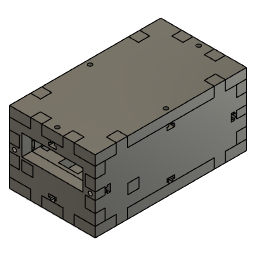
Basic-Case_v1 (Autodesk Fusion 360 design; units mm, degrees)
Autodesk Fusion 360 part; units mm, degrees
(part 1 of 2)
ref_plane "WorkPlane4" through (0, 21, 0) normal (0, 1, 0) x (0, 0, 1)
ref_plane "WorkPlane5" through (0, 0, 26.5) normal (0, 0, 1) x (1, 0, 0)
ref_plane "WorkPlane9" through (0, 0, -26.5) normal (0, 0, 1) x (1, 0, 0)
ref_plane "WorkPlane11" through (-13.285, 0, 0) normal (1, 0, 0) x (0, 1, 0)
ref_plane "WorkPlane12" through (13.285, 0, 0) normal (1, 0, 0) x (0, 1, 0)
sketch "Sketch1" plane through (0, 0, 0) normal (0, 1, 0) x (1, 0, 0)
  line L0 (12.785, -26) -> (-12.785, -26) construction
  line L1 (-12.785, -26) -> (-12.785, 26) construction
  line L2 (-12.785, 26) -> (12.785, 26) construction
  line L3 (12.785, 26) -> (12.785, -26) construction
  line L4 (12.785, -26) -> (-12.785, 26) construction
  line L5 (-12.785, -26) -> (12.785, 26) construction
  line L6 (-13.285, -26.5) -> (-13.285, 26.5)
  line L7 (-13.285, 26.5) -> (13.285, 26.5)
  line L8 (13.285, 26.5) -> (13.285, -26.5)
  line L9 (13.285, -26.5) -> (-13.285, -26.5)
  line L10 (-17.285, -30.5) -> (-17.285, 30.5)
  line L11 (-17.285, 30.5) -> (17.285, 30.5)
  line L12 (17.285, 30.5) -> (17.285, -30.5)
  line L13 (17.285, -30.5) -> (-17.285, -30.5)
  line L14 (-17.285, -22) -> (-12.785, -22)
  line L15 (-17.285, -17.5) -> (-13.285, -17.5)
  line L16 (-8.785, -26.5) -> (-8.785, -30.5)
  line L17 (-4.285, -30.5) -> (-4.285, -26.5)
  line L18 (4.285, -26.5) -> (4.285, -30.5)
  line L19 (8.785, -30.5) -> (8.785, -26.5)
  line L20 (13.285, -22) -> (17.285, -22)
  line L21 (13.285, -17.5) -> (17.285, -17.5)
  line L22 (13.285, 22) -> (17.285, 22)
  line L23 (17.285, 17.5) -> (13.285, 17.5)
  line L24 (8.785, 30.5) -> (8.785, 26.5)
  line L25 (4.285, 30.5) -> (4.285, 26.5)
  line L26 (-8.785, 30.5) -> (-8.785, 26.5)
  line L27 (-4.285, 26.5) -> (-4.285, 30.5)
  line L28 (-13.285, 22) -> (-17.285, 22)
  line L29 (-17.285, 17.5) -> (-13.285, 17.5)
  line L30 (0, -26.5) -> (0, -30.5) construction
  line L31 (13.285, 0) -> (17.285, 0) construction
  line L32 (-17.285, 0) -> (-13.285, 0) construction
  line L33 (0, 30.5) -> (0, 26.5) construction
  circle A0 centre (15.285, 0) radius 0.8
  circle A1 centre (0, 28.5) radius 0.8
  circle A2 centre (-15.285, 0) radius 0.8
  circle A3 centre (0, -28.5) radius 0.8
  dimension "d1" = 52
  dimension "d2" = 25.57
  dimension "d3" = 0.5
  dimension "d4" = 4.5
  dimension "d385" = 4.5
  dimension "d386" = 4.5
  dimension "d387" = 4.5
  dimension "d388" = 4.5
  dimension "d389" = 4.5
  dimension "d391" = 4.5
  dimension "d392" = 4.5
  dimension "d394" = 4.5
  dimension "d395" = 4.5
  dimension "d396" = 4.5
  dimension "d397" = 4.5
  dimension "d399" = 4.5
  dimension "d402" = 1.6
  dimension "d403" = 1.6
  dimension "d404" = 1.6
  dimension "d405" = 1.6
  dimension "d437" = 4.5
  dimension "d438" = 4.5
  dimension "d439" = 4.5
  dimension "d440" = 4.5
  constraint perpendicular L0 L1
  constraint parallel L0 L2
  constraint parallel L1 L3
  constraint horizontal L0
  constraint coincident L4 origin
  constraint coincident L5 origin
  constraint coincident L10 L14.start
  constraint coincident L1 L14.end
  constraint perpendicular L6 L14
  constraint coincident L10 L15.start
  constraint coincident L6 L15.end
  constraint perpendicular L1 L15
  constraint coincident L9 L16.start
  constraint coincident L13 L16.end
  constraint perpendicular L13 L16
  constraint coincident L13 L17.start
  constraint coincident L9 L17.end
  constraint perpendicular L9 L17
  constraint coincident L9 L18.start
  constraint coincident L13 L18.end
  constraint perpendicular L13 L18
  constraint coincident L13 L19.start
  constraint coincident L9 L19.end
  constraint perpendicular L0 L19
  constraint coincident L8 L20.start
  constraint coincident L12 L20.end
  constraint perpendicular L12 L20
  constraint coincident L8 L21.start
  constraint coincident L12 L21.end
  constraint perpendicular L12 L21
  constraint coincident L8 L22.start
  constraint coincident L12 L22.end
  constraint perpendicular L12 L22
  constraint coincident L12 L23.start
  constraint coincident L8 L23.end
  constraint perpendicular L8 L23
  constraint coincident L11 L24.start
  constraint coincident L7 L24.end
  constraint perpendicular L7 L24
  constraint coincident L11 L25.start
  constraint coincident L7 L25.end
  constraint perpendicular L11 L25
  constraint coincident L11 L26.start
  constraint coincident L7 L26.end
  constraint perpendicular L7 L26
  constraint coincident L7 L27.start
  constraint coincident L11 L27.end
  constraint perpendicular L11 L27
  constraint coincident L6 L28.start
  constraint coincident L10 L28.end
  constraint perpendicular L10 L28
  constraint coincident L10 L29.start
  constraint coincident L6 L29.end
  constraint perpendicular L6 L29
  constraint midpoint L9 L30.start
  constraint midpoint L13 L30.end
  constraint midpoint L8 L31.start
  constraint midpoint L12 L31.end
  constraint midpoint L10 L32.start
  constraint midpoint L6 L32.end
  constraint midpoint L11 L33.start
  constraint midpoint L7 L33.end
  constraint midpoint L31 A0.centre
  constraint midpoint L33 A1.centre
  constraint midpoint L32 A2.centre
  constraint midpoint L30 A3.centre
  measures "d1" distance of L0.start L2.end
  measures "d2" distance of L0.start L0.end
  measures "d385" distance of L28 L29
  measures "d386" distance of L26 L27
  measures "d387" distance of L6.end L26
  measures "d388" distance of L24 L25
  measures "d389" distance of L7.end L24
  measures "d391" distance of L22 L23
  measures "d392" distance of L20 L21
  measures "d394" distance of L8.end L19
  measures "d395" distance of L18 L19
  measures "d396" distance of L6.start L16
  measures "d397" distance of L16 L17
  measures "d402" diameter of A3
  measures "d403" diameter of A0
  measures "d404" diameter of A2
  measures "d405" diameter of A1
  measures "d437" distance of L6.start L14
  measures "d438" distance of L6.end L28
  measures "d439" distance of L7.end L22
  measures "d440" distance of L8.end L20
sketch "Sketch33" plane through (0, 21, 0) normal (0, 1, 0) x (1, 0, 0)
  line L0 (-17.285, 30.5) -> (17.285, 30.5)
  line L1 (-17.285, -30.5) -> (-17.285, 30.5)
  line L2 (17.285, -30.5) -> (-17.285, -30.5)
  line L3 (-13.285, -26.5) -> (-13.285, 26.5)
  line L4 (-13.285, 26.5) -> (13.285, 26.5)
  line L5 (-13.285, 22) -> (-17.285, 22)
  line L6 (-17.285, 17.5) -> (-13.285, 17.5)
  line L7 (-8.785, 30.5) -> (-8.785, 26.5)
  line L8 (-4.285, 26.5) -> (-4.285, 30.5)
  line L9 (4.285, 30.5) -> (4.285, 26.5)
  line L10 (8.785, 30.5) -> (8.785, 26.5)
  line L11 (13.285, 26.5) -> (13.285, -26.5)
  line L12 (13.285, 22) -> (17.285, 22)
  line L13 (17.285, 17.5) -> (13.285, 17.5)
  line L14 (17.285, 30.5) -> (17.285, -30.5)
  line L15 (13.285, -17.5) -> (17.285, -17.5)
  line L16 (13.285, -22) -> (17.285, -22)
  line L17 (8.785, -30.5) -> (8.785, -26.5)
  line L18 (4.285, -26.5) -> (4.285, -30.5)
  line L19 (-4.285, -30.5) -> (-4.285, -26.5)
  line L20 (-8.785, -26.5) -> (-8.785, -30.5)
  line L21 (-17.285, -22) -> (-12.785, -22)
  line L22 (-17.285, -17.5) -> (-13.285, -17.5)
  line L23 (13.285, -26.5) -> (-13.285, -26.5)
  circle A0 centre (0, -28.5) radius 0.8
  circle A1 centre (0, 28.5) radius 0.8
  circle A2 centre (-15.285, 0) radius 0.8
  circle A3 centre (15.285, 0) radius 0.8
  point P0 (15.285, 0)
  point P1 (-15.285, 0)
sketch "Sketch24" plane through (0, 0, 26.5) normal (0, 0, 1) x (1, 0, 0)
  line L0 (17.285, 0) -> (-17.285, 0)
  line L1 (17.285, 21) -> (-17.285, 21)
  line L2 (-8.785, 21) -> (-8.785, 25)
  line L3 (-4.285, 21) -> (-4.285, 25)
  line L4 (4.285, 21) -> (4.285, 25)
  line L5 (8.785, 21) -> (8.785, 25)
  line L6 (-8.785, 0) -> (-8.785, -4)
  line L7 (-4.285, 0) -> (-4.285, -4)
  line L8 (4.285, 0) -> (4.285, -4)
  line L9 (8.785, 0) -> (8.785, -4)
  line L10 (-0.8, 21) -> (-0.8, 20.1)
  line L11 (-0.8, 20.1) -> (-1.5, 20.1)
  line L12 (-1.5, 20.1) -> (-1.5, 18.9)
  line L13 (-1.5, 18.9) -> (1.5, 18.9)
  line L14 (1.5, 18.9) -> (1.5, 20.1)
  line L15 (1.5, 20.1) -> (0.8, 20.1)
  line L16 (0.8, 20.1) -> (0.8, 21)
  line L17 (-0.8, 0) -> (-0.8, 0.9)
  line L18 (-1.5, 0.9) -> (-1.5, 2.1)
  line L19 (-1.5, 2.1) -> (1.5, 2.1)
  line L20 (-0.8, 0.9) -> (-1.5, 0.9)
  line L21 (1.5, 0.9) -> (0.8, 0.9)
  line L22 (0.8, 0.9) -> (0.8, 0)
  line L23 (1.5, 2.1) -> (1.5, 0.9)
  line L24 (0, 18.9) -> (0, 21) construction
  line L25 (0, 2.1) -> (0, 0) construction
  line L26 (13.285, 16.5) -> (24.3607, 16.5)
  line L27 (13.285, 4.5) -> (17.285, 4.5)
  line L28 (-13.285, 12) -> (-17.285, 12)
  line L29 (-17.285, 9) -> (-13.285, 9)
  line L30 (-17.285, 25) -> (-17.285, -4)
  line L31 (-17.285, -4) -> (17.285, -4)
  line L32 (17.285, -4) -> (17.285, 25)
  line L33 (17.285, 25) -> (-17.285, 25)
  line L34 (-13.285, 21) -> (-13.285, 0)
  line L35 (13.285, 21) -> (13.285, 0)
  line L36 (17.285, 9) -> (13.285, 9)
  line L37 (17.285, 12) -> (13.285, 12)
  line L38 (-13.285, 16.5) -> (-17.285, 16.5)
  line L39 (-13.285, 4.5) -> (-17.285, 4.5)
  line L40 (17.285, 10.5) -> (13.285, 10.5) construction
  line L41 (-13.285, 10.5) -> (-13.285, 14.6467)
  line L42 (-17.285, 10.5) -> (-13.285, 10.5) construction
  circle A0 centre (15.285, 10.5) radius 0.8
  circle A1 centre (-15.285, 10.5) radius 0.8
  line L43 (0, 0) -> (0, 25) construction
  point P0 (-4.285, 0)
  point P1 (-8.785, 0)
  point P2 (4.285, 0)
  point P3 (8.785, 0)
  point P4 (0, 21)
  point P5 (-8.785, 21)
  point P6 (-4.285, 21)
  point P7 (8.785, 21)
  point P8 (4.285, 21)
  dimension "d406" = 3
  dimension "d407" = 1.2
  dimension "d409" = 1.6
  dimension "d410" = 1.6
  dimension "d411" = 3
  dimension "d413" = 1.2
  dimension "d420" = 6.1
  dimension "d421" = 4
  dimension "d422" = 4
  dimension "d424" = 6.1
  dimension "d425" = 4
  dimension "d426" = 4
  dimension "d427" = 4.5
  dimension "d428" = 4.5
  dimension "d429" = 4.5
  dimension "d430" = 4.5
  dimension "d433" = 4.5
  dimension "d434" = 4.5
  dimension "d435" = 1.6
  dimension "d436" = 1.6
  dimension "d482" = 4.5
  dimension "d483" = 4.5
  constraint coincident P1 L6.start
  constraint coincident P0 L7.start
  constraint coincident P2 L8.start
  constraint perpendicular L0 L8
  constraint coincident P3 L9.start
  constraint perpendicular L10 L11
  constraint perpendicular L12 L13
  constraint perpendicular L14 L15
  constraint collinear L11 L15
  constraint equal L11 L15
  constraint equal L17 L22
  constraint equal L18 L23
  constraint equal L20 L21
  constraint perpendicular L18 L19
  constraint perpendicular L19 L23
  constraint perpendicular L18 L20
  constraint perpendicular L21 L22
  constraint midpoint L13 L24.start
  constraint coincident P4 L24.end
  constraint perpendicular L1 L24
  constraint midpoint L19 L25.start
  constraint coincident L25.end L43.start
  constraint perpendicular L0 L25
  constraint perpendicular L1 L3
  constraint perpendicular L1 L2
  constraint perpendicular L1 L4
  constraint perpendicular L1 L5
  constraint vertical L30
  constraint perpendicular L32 L33
  constraint perpendicular L30 L33
  constraint perpendicular L30 L31
  constraint coincident L2.end L33
  constraint coincident L3.end L33
  constraint coincident L4.end L33
  constraint coincident L5.end L33
  constraint coincident L1.start L32
  constraint coincident L1.end L30
  constraint coincident L6.end L31
  constraint coincident L7.end L31
  constraint coincident L0 L17.start
  constraint coincident L0 L22.end
  constraint coincident L1 L10.start
  constraint coincident L1 L16.end
  constraint coincident L8.end L31
  constraint coincident L9.end L31
  constraint coincident L1 L34.start
  constraint coincident L0 L34.end
  constraint perpendicular L0 L34
  constraint coincident L1 L35.start
  constraint coincident L0 L35.end
  constraint perpendicular L0 L35
  constraint coincident L28.start L34
  constraint coincident L29.end L34
  constraint coincident L26.start L35
  constraint coincident L27.start L35
  constraint perpendicular L0 L9
  constraint perpendicular L0 L6
  constraint perpendicular L0 L7
  constraint coincident L27.end L32
  constraint perpendicular L27 L32
  constraint coincident L32 L36.start
  constraint coincident L35 L36.end
  constraint perpendicular L35 L36
  constraint coincident L32 L37.start
  constraint coincident L35 L37.end
  constraint perpendicular L35 L37
  constraint coincident L34 L38.start
  constraint coincident L30 L38.end
  constraint perpendicular L30 L38
  constraint coincident L34 L39.start
  constraint coincident L30 L39.end
  constraint perpendicular L30 L39
  constraint coincident L29.start L30
  constraint perpendicular L29 L30
  constraint midpoint L32 L40.start
  constraint midpoint L35 L40.end
  constraint midpoint L34 L41.start
  constraint coincident L34 L41.end
  constraint parallel L34 L41
  constraint midpoint L30 L42.start
  constraint midpoint L40 A0.centre
  constraint midpoint L42 A1.centre
  constraint midpoint L33 L43.end
  constraint vertical L43
  constraint equal L12 L14
  constraint coincident L1 P8
  constraint coincident L1 P7
  constraint coincident L1 P6
  constraint coincident L1 P5
  constraint coincident P5 L2.start
  constraint coincident P6 L3.start
  constraint coincident P7 L5.start
  constraint coincident P8 L4.start
  constraint coincident L0.end L30
  constraint coincident L28.end L30
  measures "d406" distance of L12.end L13.end
  measures "d407" distance of L13.end L14.end
  measures "d409" distance of L10 L16
  measures "d410" distance of L17 L22
  measures "d411" horizontal distance of L18.end L19.end
  measures "d413" distance of L18.start L18.end
  measures "d420" distance of L13 L33
  measures "d421" distance of L1 L33
  measures "d422" distance of L0 L31
  measures "d424" distance of L19 L31
  measures "d425" distance of L30 L34
  measures "d426" distance of L32 L35
  measures "d427" distance of L28 L38
  measures "d428" distance of L29 L39
  measures "d429" distance of L26 L37
  measures "d430" distance of L27 L36
  measures "d433" distance of L0 L39
  measures "d434" distance of L0.start L27
  measures "d435" diameter of A1
  measures "d436" diameter of A0
  measures "d482" distance of L1 L38
  measures "d483" distance of L1 L26
sketch "Sketch38" plane through (0, 0, -26.5) normal (0, 0, 1) x (1, 0, 0)
  line L0 (17.285, 25) -> (-17.285, 25)
  line L1 (17.285, -4) -> (17.285, 25)
  line L2 (13.285, 21) -> (13.285, 0)
  line L3 (17.285, 21) -> (-17.285, 21)
  line L4 (8.785, 21) -> (8.785, 25)
  line L5 (4.285, 21) -> (4.285, 25)
  line L6 (-4.285, 21) -> (-4.285, 25)
  line L7 (-8.785, 21) -> (-8.785, 25)
  line L8 (0.8, 20.1) -> (0.8, 21)
  line L9 (1.5, 20.1) -> (0.8, 20.1)
  line L10 (1.5, 18.9) -> (1.5, 20.1)
  line L11 (-1.5, 18.9) -> (1.5, 18.9)
  line L12 (-1.5, 20.1) -> (-1.5, 18.9)
  line L13 (-0.8, 20.1) -> (-1.5, 20.1)
  line L14 (-0.8, 21) -> (-0.8, 20.1)
  line L15 (-13.285, 21) -> (-13.285, 0)
  line L16 (-17.285, 25) -> (-17.285, -4)
  line L17 (-13.285, 16.5) -> (-17.285, 16.5)
  line L18 (-13.285, 12) -> (-17.285, 12)
  circle A0 centre (-15.285, 10.5) radius 0.8
  line L19 (-17.285, 9) -> (-13.285, 9)
  line L20 (-13.285, 4.5) -> (-17.285, 4.5)
  line L21 (17.285, 0) -> (-17.285, 0)
  line L22 (-8.785, 0) -> (-8.785, -4)
  line L23 (-17.285, -4) -> (17.285, -4)
  line L24 (-4.285, 0) -> (-4.285, -4)
  line L25 (8.785, 0) -> (8.785, -4)
  line L26 (4.285, 0) -> (4.285, -4)
  line L27 (13.285, 4.5) -> (17.285, 4.5)
  line L28 (17.285, 9) -> (13.285, 9)
  circle A1 centre (15.285, 10.5) radius 0.8
  line L29 (17.285, 12) -> (13.285, 12)
  line L30 (13.285, 16.5) -> (24.3607, 16.5)
  line L31 (-1.5, 2.1) -> (1.5, 2.1)
  line L32 (1.5, 2.1) -> (1.5, 0.9)
  line L33 (1.5, 0.9) -> (0.8, 0.9)
  line L34 (-0.8, 0.9) -> (-1.5, 0.9)
  line L35 (-0.8, 0) -> (-0.8, 0.9)
  line L36 (0.8, 0.9) -> (0.8, 0)
  line L37 (-1.5, 0.9) -> (-1.5, 2.1)
sketch "Sketch39" plane through (13.285, 0, 0) normal (1, 0, 0) x (0, 1, 0)
  line L0 (21, -30.5) -> (21, 30.5)
  line L1 (0, -30.5) -> (0, 30.5)
  line L2 (-4, 26.5) -> (25, 26.5)
  line L3 (-4, -26.5) -> (25, -26.5)
  line L4 (25, 30.5) -> (25, -30.5)
  line L5 (25, -30.5) -> (-4, -30.5)
  line L6 (-4, -30.5) -> (-4, 30.5)
  line L7 (-4, 30.5) -> (25, 30.5)
  line L8 (21, 22) -> (25, 22)
  line L9 (21, 17.5) -> (25, 17.5)
  line L10 (21, -17.5) -> (25, -17.5)
  line L11 (21, -22) -> (25, -22)
  line L12 (16.5, -26.5) -> (16.5, -30.5)
  line L13 (12, -26.5) -> (12, -30.5)
  line L14 (9, -26.5) -> (9, -30.5)
  line L15 (4.5, -26.5) -> (4.5, -30.5)
  line L16 (0, -17.5) -> (-4, -17.5)
  line L17 (0, -22) -> (-4, -22)
  line L18 (0, 22) -> (-4, 22)
  line L19 (0, 17.5) -> (-4, 17.5)
  line L20 (16.5, 26.5) -> (16.5, 30.5)
  line L21 (12, 26.5) -> (12, 30.5)
  line L22 (9, 26.5) -> (9, 30.5)
  line L23 (4.5, 26.5) -> (4.5, 30.5)
  line L24 (21, 0.8) -> (20.1, 0.8)
  line L25 (20.1, 0.8) -> (20.1, 1.5)
  line L26 (18.9, 1.5) -> (18.9, -1.5)
  line L27 (18.9, -1.5) -> (20.1, -1.5)
  line L28 (20.1, -1.5) -> (20.1, -0.8)
  line L29 (20.1, -0.8) -> (21, -0.8)
  line L30 (11.3, -26.5) -> (11.3, -25.6)
  line L31 (11.3, -25.6) -> (12, -25.6)
  line L32 (12, -25.6) -> (12, -24.4)
  line L33 (12, -24.4) -> (9, -24.4)
  line L34 (9, -24.4) -> (9, -25.6)
  line L35 (9, -25.6) -> (9.7, -25.6)
  line L36 (9.7, -25.6) -> (9.7, -26.5)
  line L37 (0, 0.8) -> (0.9, 0.8)
  line L38 (0.9, 0.8) -> (0.9, 1.5)
  line L39 (0.9, 1.5) -> (2.1, 1.5)
  line L40 (2.1, 1.5) -> (2.1, -1.5)
  line L41 (2.1, -1.5) -> (0.9, -1.5)
  line L42 (0.9, -1.5) -> (0.9, -0.8)
  line L43 (0.9, -0.8) -> (0, -0.8)
  line L44 (9.7, 26.5) -> (9.7, 25.6)
  line L45 (9.7, 25.6) -> (9, 25.6)
  line L46 (9, 25.6) -> (9, 24.4)
  line L47 (9, 24.4) -> (12, 24.4)
  line L48 (12, 24.4) -> (12, 25.6)
  line L49 (12, 25.6) -> (11.3, 25.6)
  line L50 (11.3, 25.6) -> (11.3, 26.5)
  line L51 (10.5, 26.5) -> (10.5, 24.4) construction
  line L52 (25, 0) -> (18.9, 0) construction
  line L53 (10.5, -24.4) -> (10.5, -30.5) construction
  line L54 (-4, 0) -> (2.1, 0) construction
  line L55 (20.1, 1.5) -> (18.9, 1.5)
  point P0 (21, 22)
  point P1 (21, 17.5)
  point P2 (21, -17.5)
  point P3 (21, -22)
  point P4 (0, -22)
  point P5 (0, 17.5)
  point P6 (21, 0)
  point P7 (0, -17.5)
  point P8 (0, 22)
  point P9 (9, 26.5)
  point P10 (4.5, 26.5)
  point P11 (16.5, 26.5)
  point P12 (12, 26.5)
  point P13 (21, 26.5)
  point P14 (16.5, -26.5)
  point P15 (12, -26.5)
  point P16 (9, -26.5)
  point P17 (4.5, -26.5)
  point P18 (10.5, -26.5)
  point P19 (10.5, 26.5)
  dimension "d452" = 1.2
  dimension "d453" = 3
  dimension "d454" = 1.6
  dimension "d455" = 6.1
  dimension "d456" = 3
  dimension "d457" = 1.6
  dimension "d458" = 1.2
  dimension "d459" = 6.1
  dimension "d460" = 1.6
  dimension "d461" = 3
  dimension "d462" = 1.2
  dimension "d463" = 6.1
  dimension "d464" = 1.2
  dimension "d465" = 1.6
  dimension "d466" = 3
  dimension "d467" = 6.1
  constraint perpendicular L2 L4
  constraint perpendicular L4 L5
  constraint perpendicular L5 L6
  constraint coincident L2.end L4
  constraint coincident L0.end L7
  constraint coincident L1.end L7
  constraint coincident L2.start L6
  constraint coincident L1.start L5
  constraint coincident P0 L8.start
  constraint coincident L4 L8.end
  constraint perpendicular L4 L8
  constraint coincident P1 L9.start
  constraint coincident L4 L9.end
  constraint perpendicular L4 L9
  constraint coincident P2 L10.start
  constraint coincident L4 L10.end
  constraint perpendicular L4 L10
  constraint coincident P3 L11.start
  constraint coincident L4 L11.end
  constraint perpendicular L4 L11
  constraint coincident P14 L12.start
  constraint coincident L5 L12.end
  constraint perpendicular L5 L12
  constraint coincident P15 L13.start
  constraint coincident L5 L13.end
  constraint perpendicular L5 L13
  constraint coincident P16 L14.start
  constraint coincident L5 L14.end
  constraint perpendicular L5 L14
  constraint coincident P17 L15.start
  constraint coincident L5 L15.end
  constraint perpendicular L5 L15
  constraint coincident P7 L16.start
  constraint coincident L6 L16.end
  constraint perpendicular L6 L16
  constraint coincident P4 L17.start
  constraint coincident L6 L17.end
  constraint perpendicular L6 L17
  constraint coincident P8 L18.start
  constraint coincident L6 L18.end
  constraint perpendicular L6 L18
  constraint coincident P5 L19.start
  constraint coincident L6 L19.end
  constraint perpendicular L6 L19
  constraint coincident P11 L20.start
  constraint coincident L7 L20.end
  constraint perpendicular L7 L20
  constraint coincident P12 L21.start
  constraint coincident L7 L21.end
  constraint perpendicular L7 L21
  constraint coincident P9 L22.start
  constraint coincident L7 L22.end
  constraint perpendicular L7 L22
  constraint coincident P10 L23.start
  constraint coincident L7 L23.end
  constraint perpendicular L7 L23
  constraint coincident L0 L24.start
  constraint perpendicular L0 L24
  constraint perpendicular L24 L25
  constraint perpendicular L26 L27
  constraint perpendicular L27 L28
  constraint coincident L0 L29.end
  constraint perpendicular L0 L29
  constraint coincident L3 L30.start
  constraint perpendicular L3 L30
  constraint perpendicular L30 L31
  constraint perpendicular L3 L32
  constraint perpendicular L32 L33
  constraint perpendicular L33 L34
  constraint perpendicular L32 L35
  constraint coincident L3 L36.end
  constraint perpendicular L3 L36
  constraint coincident L1 L37.start
  constraint perpendicular L1 L37
  constraint perpendicular L37 L38
  constraint perpendicular L38 L39
  constraint perpendicular L39 L40
  constraint perpendicular L38 L41
  constraint perpendicular L39 L42
  constraint coincident L1 L43.end
  constraint perpendicular L1 L43
  constraint coincident L2 L44.start
  constraint perpendicular L2 L44
  constraint perpendicular L44 L45
  constraint perpendicular L2 L46
  constraint perpendicular L44 L47
  constraint perpendicular L47 L48
  constraint perpendicular L48 L49
  constraint coincident L2 L50.end
  constraint perpendicular L2 L50
  constraint coincident P19 L51.start
  constraint midpoint L47 L51.end
  constraint midpoint L4 L52.start
  constraint midpoint L26 L52.end
  constraint midpoint L33 L53.start
  constraint midpoint L5 L53.end
  constraint midpoint L6 L54.start
  constraint midpoint L40 L54.end
  constraint vertical L53
  constraint horizontal L52
  constraint vertical L51
  constraint horizontal L54
  constraint equal L38 L42
  constraint equal L37 L43
  constraint equal L24 L29
  constraint equal L25 L28
  constraint equal L44 L50
  constraint equal L45 L49
  constraint equal L31 L35
  constraint equal L30 L36
  constraint perpendicular L26 L55
  constraint vertical L26
  measures "d452" distance of L31.end L32.end
  measures "d453" distance of L32.end L33.end
  measures "d454" distance of L30 L36
  measures "d455" distance of L5 L33
  measures "d456" distance of L26.start L26.end
  measures "d457" distance of L24 L29
  measures "d458" distance of L26.end L27.end
  measures "d459" distance of L4 L26
  measures "d460" distance of L44 L50
  measures "d461" distance of L46.end L47.end
  measures "d462" distance of L47.end L48.end
  measures "d463" distance of L7 L47
  measures "d464" distance of L38.end L39.end
  measures "d465" distance of L37 L43
  measures "d466" distance of L39.end L40.end
  measures "d467" distance of L6 L40
sketch "Sketch40" plane through (-13.285, 0, 0) normal (1, 0, 0) x (0, 1, 0)
  line L0 (25, 30.5) -> (25, -30.5)
  line L1 (25, -30.5) -> (-4, -30.5)
  line L2 (-4, -26.5) -> (25, -26.5)
  line L3 (21, -30.5) -> (21, 30.5)
  line L4 (21, -22) -> (25, -22)
  line L5 (21, -17.5) -> (25, -17.5)
  line L6 (16.5, -26.5) -> (16.5, -30.5)
  line L7 (12, -26.5) -> (12, -30.5)
  line L8 (9, -26.5) -> (9, -30.5)
  line L9 (4.5, -26.5) -> (4.5, -30.5)
  line L10 (-4, -30.5) -> (-4, 30.5)
  line L11 (0, -30.5) -> (0, 30.5)
  line L12 (0, -22) -> (-4, -22)
  line L13 (0, -17.5) -> (-4, -17.5)
  line L14 (0, 17.5) -> (-4, 17.5)
  line L15 (0, 22) -> (-4, 22)
  line L16 (-4, 26.5) -> (25, 26.5)
  line L17 (9, 26.5) -> (9, 30.5)
  line L18 (4.5, 26.5) -> (4.5, 30.5)
  line L19 (12, 26.5) -> (12, 30.5)
  line L20 (16.5, 26.5) -> (16.5, 30.5)
  line L21 (21, 17.5) -> (25, 17.5)
  line L22 (21, 22) -> (25, 22)
  line L23 (20.1, -0.8) -> (21, -0.8)
  line L24 (20.1, -1.5) -> (20.1, -0.8)
  line L25 (18.9, -1.5) -> (20.1, -1.5)
  line L26 (18.9, 1.5) -> (18.9, -1.5)
  line L27 (20.1, 1.5) -> (18.9, 1.5)
  line L28 (20.1, 0.8) -> (20.1, 1.5)
  line L29 (21, 0.8) -> (20.1, 0.8)
  line L30 (11.3, -26.5) -> (11.3, -25.6)
  line L31 (12, -25.6) -> (12, -24.4)
  line L32 (12, -24.4) -> (9, -24.4)
  line L33 (11.3, -25.6) -> (12, -25.6)
  line L34 (9, -24.4) -> (9, -25.6)
  line L35 (9, -25.6) -> (9.7, -25.6)
  line L36 (9.7, -25.6) -> (9.7, -26.5)
  line L37 (2.1, -1.5) -> (0.9, -1.5)
  line L38 (2.1, 1.5) -> (2.1, -1.5)
  line L39 (0.9, 1.5) -> (2.1, 1.5)
  line L40 (0.9, 0.8) -> (0.9, 1.5)
  line L41 (0, 0.8) -> (0.9, 0.8)
  line L42 (0.9, -0.8) -> (0, -0.8)
  line L43 (0.9, -1.5) -> (0.9, -0.8)
  line L44 (9, 24.4) -> (12, 24.4)
  line L45 (12, 24.4) -> (12, 25.6)
  line L46 (12, 25.6) -> (11.3, 25.6)
  line L47 (11.3, 25.6) -> (11.3, 26.5)
  line L48 (9.7, 26.5) -> (9.7, 25.6)
  line L49 (9.7, 25.6) -> (9, 25.6)
  line L50 (9, 25.6) -> (9, 24.4)
  line L51 (-4, 30.5) -> (25, 30.5)
extrude "Extrude52" add sketch "Sketch1" against normal blind 4 contours L6 L10 L15 L29 | L6 L7 L8 L9 | L6 L9 L10 L13 L14 L16 | L6 L7 L10 L11 L26 L28 | L9 L13 L17 L18 | L7 L11 L25 L27 | L8 L9 L12 L13 L19 L20 | L7 L8 L11 L12 L22 L24 | L8 L12 L21 L23 makes body 1
extrude "Extrude53" add sketch "Sketch33" along normal blind 4 separate body contours L0 L1 L3 L4 L5 L7 | L0 L4 L8 L9 | L3 L4 L11 L23 | L1 L3 L6 L22 | L0 L4 L10 L11 L12 L14 | L1 L2 L3 L20 L21 L23 | L11 L13 L14 L15 | L2 L18 L19 L23 | L2 L11 L14 L16 L17 L23 makes body 2
extrude "Extrude54" add sketch "Sketch24" along normal blind 4 separate body contours L0 L27 L32 L35 | L0 L1 L10 L11 L12 L13 L14 L15 L16 L17 L18 L19 L20 L21 L22 L23 L34 L35 L41 | L0 L8 L9 L31 | L32 L35 L36 L37 | L0 L6 L7 L31 | L1 L26 L32 L35 | L1 L4 L5 L33 | L0 L30 L34 L39 | L28 L29 L30 L34 L41 | L1 L2 L3 L33 | L1 L30 L34 L38 makes body 3
extrude "Extrude55" add sketch "Sketch38" against normal blind 4 separate body contours L0 L3 L4 L5 | L1 L2 L3 L30 | L2 L3 L8 L9 L10 L11 L12 L13 L14 L15 L21 L31 L32 L33 L34 L35 L36 L37 | L0 L3 L6 L7 | L1 L2 L28 L29 | L1 L2 L21 L27 | L3 L15 L16 L17 | L15 L16 L18 L19 | L21 L23 L25 L26 | L15 L16 L20 L21 | L21 L22 L23 L24 makes body 4
extrude "Extrude56" add sketch "Sketch39" along normal blind 4 separate body contours L0 L1 L2 L3 L24 L25 L26 L27 L28 L29 L30 L31 L32 L33 L34 L35 L36 L37 L38 L39 L40 L41 L42 L43 L44 L45 L46 L47 L48 L49 L50 L55 | L0 L4 L10 L11 | L3 L5 L12 L13 | L0 L4 L8 L9 | L3 L5 L14 L15 | L2 L7 L20 L21 | L1 L6 L16 L17 | L2 L7 L22 L23 | L1 L6 L18 L19 makes body 5
extrude "Extrude57" add sketch "Sketch40" against normal blind 4 separate body contours L0 L3 L21 L22 | L2 L3 L11 L16 L23 L24 L25 L26 L27 L28 L29 L30 L31 L32 L33 L34 L35 L36 L37 L38 L39 L40 L41 L42 L43 L44 L45 L46 L47 L48 L49 L50 | L16 L19 L20 L51 | L0 L3 L4 L5 | L16 L17 L18 L51 | L1 L2 L6 L7 | L10 L11 L14 L15 | L1 L2 L8 L9 | L10 L11 L12 L13 makes body 6
ref_plane "WorkPlane13" through (0, 4.5, 0) normal (0, 1, 0) x (0, 0, 1)
sketch "Sketch41" plane through (0, 4.5, 0) normal (0, 1, 0) x (1, 0, 0)
  line L0 (-13.285, -26.5) -> (-13.285, 26.5)
  line L1 (-13.285, 26.5) -> (13.285, 26.5)
  line L2 (13.285, 26.5) -> (13.285, -26.5)
  line L3 (13.285, -26.5) -> (-13.285, -26.5)
  line L4 (-17.285, -17.5) -> (-13.285, -17.5) construction
  line L5 (17.285, 30.5) -> (17.285, -30.5)
  line L6 (-17.285, 30.5) -> (17.285, 30.5)
  line L7 (-17.285, -30.5) -> (-17.285, 30.5)
  line L8 (17.285, -30.5) -> (-17.285, -30.5)
  line L9 (-17.285, 17.35) -> (-13.285, 17.35)
  line L10 (-17.285, 12.85) -> (-13.285, 12.85)
  line L11 (7.85, 26.5) -> (7.85, 30.5)
  line L12 (12.35, 26.5) -> (12.35, 30.5)
  line L13 (13.285, -12.85) -> (17.285, -12.85)
  line L14 (13.285, -17.35) -> (17.285, -17.35)
  line L15 (-7.85, -26.5) -> (-7.85, -30.5)
  line L16 (-12.35, -26.5) -> (-12.35, -30.5)
  circle A0 centre (0, 28.5) radius 0.8 construction
  circle A1 centre (15.285, 0) radius 0.8 construction
  circle A2 centre (-15.285, 0) radius 0.8 construction
  circle A3 centre (0, -28.5) radius 0.8 construction
  line L17 (-12.35, -26.5) -> (-7.85, -30.5) construction
  line L18 (13.285, -17.35) -> (17.285, -12.85) construction
  line L19 (7.85, 30.5) -> (12.35, 26.5) construction
  line L20 (-17.285, 17.35) -> (-13.285, 12.85) construction
  line L21 (-20.2, -28.5) -> (0, -28.5) construction
  line L22 (15.285, -30.2) -> (15.285, 0) construction
  line L23 (-15.285, 0) -> (-15.285, 30.2) construction
  line L24 (0, 28.5) -> (20.2, 28.5) construction
  line L25 (13.285, 26.5) -> (13.285, 30.5) construction
  line L26 (-13.285, 26.5) -> (-17.285, 26.5) construction
  line L27 (-13.285, -26.5) -> (-13.285, -30.5) construction
  line L28 (13.285, -26.5) -> (17.285, -26.5) construction
  point P0 (0, -28.5)
  dimension "d474" = 4.5
  dimension "d475" = 4.5
  dimension "d476" = 4.5
  dimension "d477" = 4.5
  constraint coincident L7 L9.start
  constraint coincident L0 L9.end
  constraint perpendicular L0 L9
  constraint coincident L7 L10.start
  constraint coincident L0 L10.end
  constraint perpendicular L0 L10
  constraint coincident L1 L11.start
  constraint coincident L6 L11.end
  constraint perpendicular L6 L11
  constraint coincident L1 L12.start
  constraint coincident L6 L12.end
  constraint perpendicular L6 L12
  constraint coincident L2 L13.start
  constraint coincident L5 L13.end
  constraint perpendicular L5 L13
  constraint coincident L2 L14.start
  constraint coincident L5 L14.end
  constraint perpendicular L5 L14
  constraint coincident L3 L15.start
  constraint coincident L8 L15.end
  constraint perpendicular L8 L15
  constraint coincident L3 L16.start
  constraint coincident L8 L16.end
  constraint perpendicular L8 L16
  constraint coincident P0 A3.centre
  constraint coincident A1.centre L22.end
  constraint coincident A2.centre L23.start
  constraint coincident A0.centre L24.start
  constraint midpoint L17 L21
  constraint midpoint L18 L22
  constraint midpoint L20 L23
  constraint midpoint L19 L24
  constraint coincident L1.end L2.start
  constraint coincident L6 L25.end
  constraint perpendicular L6 L25
  constraint coincident L0.end L1.start
  constraint coincident L7 L26.end
  constraint perpendicular L7 L26
  constraint coincident L0.start L3.end
  constraint coincident L8 L27.end
  constraint perpendicular L8 L27
  constraint coincident L2.end L3.start
  constraint coincident L5 L28.end
  constraint perpendicular L5 L28
  constraint perpendicular L22 L28
  constraint perpendicular L21 L27
  constraint perpendicular L23 L26
  measures "d474" distance of L9 L10
  measures "d475" distance of L11 L12
  measures "d476" distance of L13 L14
  measures "d477" distance of L15 L16
extrude "Extrude59" cut sketch "Sketch41" along normal blind 4 contours L0 L7 L9 L10 | L3 L8 L15 L16 | L1 L6 L11 L12 | L2 L5 L13 L14 bodies 3 4 5 6
extrude "Extrude58" add sketch "Sketch41" along normal blind 4 separate body contours L0 L1 L2 L3 | L0 L7 L9 L10 | L3 L8 L15 L16 | L1 L6 L11 L12 | L2 L5 L13 L14 makes body 7
ref_plane "WorkPlane15" through (0, 8.5, 0) normal (0, 1, 0) x (0, 0, 1)
sketch "Sketch45" plane through (0, 8.5, 0) normal (0, 1, 0) x (1, 0, 0)
  line L0 (12.785, -22.32) -> (10.265, -22.32)
  line L1 (10.265, -22.32) -> (10.265, 23.52)
  line L2 (10.265, 23.52) -> (12.785, 23.52)
  line L3 (12.785, 23.52) -> (12.785, -22.32)
  line L4 (13.285, -12.85) -> (13.285, 26.5)
  line L5 (-12.785, -22.32) -> (-10.265, -22.32)
  line L6 (-10.265, -22.32) -> (-10.265, 23.52)
  line L7 (-10.265, 23.52) -> (-12.785, 23.52)
  line L8 (-12.785, 23.52) -> (-12.785, -22.32)
  line L9 (-13.285, 12.85) -> (-13.285, -26.5)
  line L10 (7.85, 26.5) -> (12.35, 26.5)
  line L11 (7.85, 26.5) -> (-13.285, 26.5)
  line L12 (-3.91, -24.1297) -> (3.89, -24.1297)
  line L13 (3.89, -24.1297) -> (3.89, -10.1297)
  line L14 (3.89, -10.1297) -> (-3.91, -10.1297)
  line L15 (-3.91, -10.1297) -> (-3.91, -24.1297)
  dimension "d489" = 2.52
  dimension "d490" = 45.84
  dimension "d491" = 0.5
  dimension "d492" = 2.52
  dimension "d493" = 45.84
  dimension "d494" = 0.5
  dimension "d496" = 2.98
  dimension "d497" = 2.98
  dimension "d500" = 7.8
  dimension "d501" = 14
  constraint horizontal L0
  constraint vertical L1
  constraint horizontal L2
  constraint vertical L3
  constraint horizontal L5
  constraint vertical L6
  constraint horizontal L7
  constraint vertical L8
  constraint horizontal L12
  constraint vertical L13
  constraint horizontal L14
  constraint vertical L15
  measures "d489" distance of L0.start L0.end
  measures "d490" distance of L0.end L1.end
  measures "d491" distance of L3 L4
  measures "d492" distance of L5.start L5.end
  measures "d493" distance of L5.start L7.end
  measures "d494" distance of L8 L9
  measures "d496" distance of L2 L10
  measures "d497" distance of L7 L11
  measures "d500" distance of L12.start L12.end
  measures "d501" distance of L12.start L14.end
extrude "Extrude60" cut sketch "Sketch45" against normal blind 22 contours L0 L1 L2 L3 | L5 L6 L7 L8 bodies 1 7
extrude "Extrude61" cut sketch "Sketch45" against normal up to surface (4 mm away) contours L12 L13 L14 L15 bodies 7
ref_plane "WorkPlane16" through (0, 10.5, 30.5) normal (0, 0, 1) x (1, 0, 0)
sketch "Sketch46" plane through (0, 10.4, 30.5) normal (0, 0, 1) x (1, 0, 0)
  line L0 (-12.285, -0.9) -> (12.285, -0.9)
  line L1 (12.285, -0.9) -> (12.285, 7.5)
  line L2 (12.285, 7.5) -> (-12.285, 7.5)
  line L3 (-12.285, 7.5) -> (-12.285, -0.9)
  line L4 (-13.285, 6.1) -> (-13.285, 1.6)
  line L5 (13.285, 1.6) -> (13.285, 6.1)
  line L6 (1.5, 8.5) -> (-1.5, 8.5)
  line L7 (-12.35, -1.9) -> (-7.85, -1.9)
  dimension "d508" = 1
  dimension "d509" = 1
  dimension "d510" = 1
  dimension "d513" = 1
  constraint horizontal L0
  constraint vertical L1
  constraint horizontal L2
  constraint vertical L3
  measures "d508" distance of L3 L4
  measures "d509" distance of L1 L5
  measures "d510" distance of L2 L6
  measures "d513" distance of L0 L7
extrude "Extrude62" cut sketch "Sketch46" against normal up to surface (4 mm away) bodies 3
sketch "Top" plane through (0, 29.4, 0) normal (0, 1, 0) x (-1, 0, 0) in component "DXF Export"
  circle A0 centre (0, 32.2) radius 0.8
  circle A1 centre (22.2, 0) radius 0.8
  circle A2 centre (-22.2, 0) radius 0.8
  circle A3 centre (0, -32.2) radius 0.8
  line L0 (-20.2, 21.2) -> (-24.2, 21.2)
  line L1 (-24.2, 21.2) -> (-24.2, -21.2)
  line L2 (-24.2, -21.2) -> (-20.2, -21.2)
  line L3 (-20.2, -21.2) -> (-20.2, -25.7)
  line L4 (-20.2, -25.7) -> (-24.2, -25.7)
  line L5 (-24.2, -25.7) -> (-24.2, -34.2)
  line L6 (-24.2, -34.2) -> (-15.7, -34.2)
  line L7 (-15.7, -34.2) -> (-15.7, -30.2)
  line L8 (-15.7, -30.2) -> (-11.2, -30.2)
  line L9 (-11.2, -30.2) -> (-11.2, -34.2)
  line L10 (-11.2, -34.2) -> (11.2, -34.2)
  line L11 (11.2, -34.2) -> (11.2, -30.2)
  line L12 (11.2, -30.2) -> (15.7, -30.2)
  line L13 (15.7, -30.2) -> (15.7, -34.2)
  line L14 (15.7, -34.2) -> (24.2, -34.2)
  line L15 (24.2, -34.2) -> (24.2, -25.7)
  line L16 (24.2, -25.7) -> (20.2, -25.7)
  line L17 (20.2, -25.7) -> (20.2, -21.2)
  line L18 (20.2, -21.2) -> (24.2, -21.2)
  line L19 (24.2, -21.2) -> (24.2, 21.2)
  line L20 (24.2, 21.2) -> (20.2, 21.2)
  line L21 (20.2, 21.2) -> (20.2, 25.7)
  line L22 (20.2, 25.7) -> (24.2, 25.7)
  line L23 (24.2, 25.7) -> (24.2, 34.2)
  line L24 (24.2, 34.2) -> (15.7, 34.2)
  line L25 (15.7, 34.2) -> (15.7, 30.2)
  line L26 (15.7, 30.2) -> (11.2, 30.2)
  line L27 (11.2, 30.2) -> (11.2, 34.2)
  line L28 (11.2, 34.2) -> (-11.2, 34.2)
  line L29 (-11.2, 34.2) -> (-11.2, 30.2)
  line L30 (-11.2, 30.2) -> (-15.7, 30.2)
  line L31 (-15.7, 30.2) -> (-15.7, 34.2)
  line L32 (-15.7, 34.2) -> (-24.2, 34.2)
  line L33 (-24.2, 34.2) -> (-24.2, 25.7)
  line L34 (-24.2, 25.7) -> (-20.2, 25.7)
  line L35 (-20.2, 25.7) -> (-20.2, 21.2)
sketch "Bottom" plane through (0, -4, 0) normal (0, -1, 0) x (1, 0, 0) in component "DXF Export"
  circle A0 centre (0, 32.2) radius 0.8
  circle A1 centre (-22.2, 0) radius 0.8
  circle A2 centre (0, -32.2) radius 0.8
  circle A3 centre (22.2, 0) radius 0.8
  line L0 (-20.2, 21.2) -> (-24.2, 21.2)
  line L1 (-24.2, 21.2) -> (-24.2, -21.2)
  line L2 (-24.2, -21.2) -> (-20.2, -21.2)
  line L3 (-20.2, -21.2) -> (-20.2, -25.7)
  line L4 (-20.2, -25.7) -> (-24.2, -25.7)
  line L5 (-24.2, -25.7) -> (-24.2, -34.2)
  line L6 (-24.2, -34.2) -> (-15.7, -34.2)
  line L7 (-15.7, -34.2) -> (-15.7, -30.2)
  line L8 (-15.7, -30.2) -> (-11.2, -30.2)
  line L9 (-11.2, -30.2) -> (-11.2, -34.2)
  line L10 (-11.2, -34.2) -> (11.2, -34.2)
  line L11 (11.2, -34.2) -> (11.2, -30.2)
  line L12 (11.2, -30.2) -> (15.7, -30.2)
  line L13 (15.7, -30.2) -> (15.7, -34.2)
  line L14 (15.7, -34.2) -> (24.2, -34.2)
  line L15 (24.2, -34.2) -> (24.2, -25.7)
  line L16 (24.2, -25.7) -> (20.2, -25.7)
  line L17 (20.2, -25.7) -> (20.2, -21.2)
  line L18 (20.2, -21.2) -> (24.2, -21.2)
  line L19 (24.2, -21.2) -> (24.2, 21.2)
  line L20 (24.2, 21.2) -> (20.2, 21.2)
  line L21 (20.2, 21.2) -> (20.2, 25.7)
  line L22 (20.2, 25.7) -> (24.2, 25.7)
  line L23 (24.2, 25.7) -> (24.2, 34.2)
  line L24 (24.2, 34.2) -> (15.7, 34.2)
  line L25 (15.7, 34.2) -> (15.7, 30.2)
  line L26 (15.7, 30.2) -> (11.2, 30.2)
  line L27 (11.2, 30.2) -> (11.2, 34.2)
  line L28 (11.2, 34.2) -> (-11.2, 34.2)
  line L29 (-11.2, 34.2) -> (-11.2, 30.2)
  line L30 (-11.2, 30.2) -> (-15.7, 30.2)
  line L31 (-15.7, 30.2) -> (-15.7, 34.2)
  line L32 (-15.7, 34.2) -> (-24.2, 34.2)
  line L33 (-24.2, 34.2) -> (-24.2, 25.7)
  line L34 (-24.2, 25.7) -> (-20.2, 25.7)
  line L35 (-20.2, 25.7) -> (-20.2, 21.2)
sketch "Front" plane through (0, 0, 34.2) normal (0, 0, 1) x (1, 0, 0) in component "DXF Export"
  line L0 (-12.35, 5.2) -> (-12.35, 9.2)
  line L1 (-12.35, 9.2) -> (-7.85, 9.2)
  line L2 (-7.85, 9.2) -> (-7.85, 5.2)
  line L3 (-7.85, 5.2) -> (-12.35, 5.2)
  circle A0 centre (22.2, 12.7) radius 0.8
  circle A1 centre (-22.2, 12.7) radius 0.8
  line L4 (-24.2, 16.4) -> (-24.2, 9)
  line L5 (-24.2, 9) -> (-20.2, 9)
  line L6 (-20.2, 9) -> (-20.2, 4.5)
  line L7 (-20.2, 4.5) -> (-24.2, 4.5)
  line L8 (-24.2, 4.5) -> (-24.2, 0)
  line L9 (-24.2, 0) -> (-15.7, 0)
  line L10 (-15.7, 0) -> (-15.7, -4)
  line L11 (-15.7, -4) -> (-11.2, -4)
  line L12 (-11.2, -4) -> (-11.2, 0)
  line L13 (-11.2, 0) -> (-0.8, 0)
  line L14 (-0.8, 0) -> (-0.8, 0.9)
  line L15 (-0.8, 0.9) -> (-1.5, 0.9)
  line L16 (-1.5, 0.9) -> (-1.5, 2.1)
  line L17 (-1.5, 2.1) -> (1.5, 2.1)
  line L18 (1.5, 2.1) -> (1.5, 0.9)
  line L19 (1.5, 0.9) -> (0.8, 0.9)
  line L20 (0.8, 0.9) -> (0.8, 0)
  line L21 (0.8, 0) -> (11.2, 0)
  line L22 (11.2, 0) -> (11.2, -4)
  line L23 (11.2, -4) -> (15.7, -4)
  line L24 (15.7, -4) -> (15.7, 0)
  line L25 (15.7, 0) -> (24.2, 0)
  line L26 (24.2, 0) -> (24.2, 4.5)
  line L27 (24.2, 4.5) -> (20.2, 4.5)
  line L28 (20.2, 4.5) -> (20.2, 9)
  line L29 (20.2, 9) -> (24.2, 9)
  line L30 (24.2, 9) -> (24.2, 16.4)
  line L31 (24.2, 25.4) -> (15.7, 25.4)
  line L32 (15.7, 25.4) -> (15.7, 29.4)
  line L33 (15.7, 29.4) -> (11.2, 29.4)
  line L34 (11.2, 29.4) -> (11.2, 25.4)
  line L35 (11.2, 25.4) -> (0.8, 25.4)
  line L36 (0.8, 25.4) -> (0.8, 24.5)
  line L37 (0.8, 24.5) -> (1.5, 24.5)
  line L38 (1.5, 24.5) -> (1.5, 23.3)
  line L39 (1.5, 23.3) -> (-1.5, 23.3)
  line L40 (-1.5, 23.3) -> (-1.5, 24.5)
  line L41 (-1.5, 24.5) -> (-0.8, 24.5)
  line L42 (-0.8, 24.5) -> (-0.8, 25.4)
  line L43 (-0.8, 25.4) -> (-11.2, 25.4)
  line L44 (-11.2, 25.4) -> (-11.2, 29.4)
  line L45 (-11.2, 29.4) -> (-15.7, 29.4)
  line L46 (-15.7, 29.4) -> (-15.7, 25.4)
  line L47 (-15.7, 25.4) -> (-24.2, 25.4)
  line L48 (-20.2, 20.9) -> (-20.2, 16.4)
  line L49 (-20.2, 16.4) -> (-24.2, 16.4)
  line L50 (24.2, 16.4) -> (20.2, 16.4)
  line L51 (20.2, 16.4) -> (20.2, 20.9)
  line L52 (20.2, 20.9) -> (24.2, 20.9)
  line L53 (24.2, 20.9) -> (24.2, 25.4)
  line L54 (-24.2, 25.4) -> (-24.2, 20.9)
  line L55 (-24.2, 20.9) -> (-20.2, 20.9)
sketch "Back" plane through (0, 0, -34.2) normal (0, 0, -1) x (-1, 0, 0) in component "DXF Export"
  line L0 (-12.35, 5.2) -> (-12.35, 9.2)
  line L1 (-12.35, 9.2) -> (-7.85, 9.2)
  line L2 (-7.85, 9.2) -> (-7.85, 5.2)
  line L3 (-7.85, 5.2) -> (-12.35, 5.2)
  circle A0 centre (22.2, 12.7) radius 0.8
  circle A1 centre (-22.2, 12.7) radius 0.8
  line L4 (0.8, 0.9) -> (0.8, 0)
  line L5 (0.8, 0) -> (11.2, 0)
  line L6 (11.2, 0) -> (11.2, -4)
  line L7 (11.2, -4) -> (15.7, -4)
  line L8 (15.7, -4) -> (15.7, 0)
  line L9 (15.7, 0) -> (24.2, 0)
  line L10 (24.2, 0) -> (24.2, 4.5)
  line L11 (24.2, 4.5) -> (20.2, 4.5)
  line L12 (20.2, 4.5) -> (20.2, 9)
  line L13 (20.2, 9) -> (24.2, 9)
  line L14 (24.2, 9) -> (24.2, 16.4)
  line L15 (24.2, 25.4) -> (15.7, 25.4)
  line L16 (15.7, 25.4) -> (15.7, 29.4)
  line L17 (15.7, 29.4) -> (11.2, 29.4)
  line L18 (11.2, 29.4) -> (11.2, 25.4)
  line L19 (11.2, 25.4) -> (0.8, 25.4)
  line L20 (0.8, 25.4) -> (0.8, 24.5)
  line L21 (0.8, 24.5) -> (1.5, 24.5)
  line L22 (1.5, 24.5) -> (1.5, 23.3)
  line L23 (1.5, 23.3) -> (-1.5, 23.3)
  line L24 (-1.5, 23.3) -> (-1.5, 24.5)
  line L25 (-1.5, 24.5) -> (-0.8, 24.5)
  line L26 (-0.8, 24.5) -> (-0.8, 25.4)
  line L27 (-0.8, 25.4) -> (-11.2, 25.4)
  line L28 (-11.2, 25.4) -> (-11.2, 29.4)
  line L29 (-11.2, 29.4) -> (-15.7, 29.4)
  line L30 (-15.7, 29.4) -> (-15.7, 25.4)
  line L31 (-15.7, 25.4) -> (-24.2, 25.4)
  line L32 (-24.2, 16.4) -> (-24.2, 9)
  line L33 (-24.2, 9) -> (-20.2, 9)
  line L34 (-20.2, 9) -> (-20.2, 4.5)
  line L35 (-20.2, 4.5) -> (-24.2, 4.5)
  line L36 (-24.2, 4.5) -> (-24.2, 0)
  line L37 (-24.2, 0) -> (-15.7, 0)
  line L38 (-15.7, 0) -> (-15.7, -4)
  line L39 (-15.7, -4) -> (-11.2, -4)
  line L40 (-11.2, -4) -> (-11.2, 0)
  line L41 (-11.2, 0) -> (-0.8, 0)
  line L42 (-0.8, 0) -> (-0.8, 0.9)
  line L43 (-0.8, 0.9) -> (-1.5, 0.9)
  line L44 (-1.5, 0.9) -> (-1.5, 2.1)
  line L45 (-1.5, 2.1) -> (1.5, 2.1)
  line L46 (1.5, 2.1) -> (1.5, 0.9)
  line L47 (1.5, 0.9) -> (0.8, 0.9)
  line L48 (24.2, 16.4) -> (20.2, 16.4)
  line L49 (20.2, 16.4) -> (20.2, 20.9)
  line L50 (20.2, 20.9) -> (24.2, 20.9)
  line L51 (24.2, 20.9) -> (24.2, 25.4)
  line L52 (-24.2, 25.4) -> (-24.2, 20.9)
  line L53 (-24.2, 20.9) -> (-20.2, 20.9)
  line L54 (-20.2, 20.9) -> (-20.2, 16.4)
  line L55 (-20.2, 16.4) -> (-24.2, 16.4)
sketch "Right" plane through (24.2, 0, 0) normal (1, 0, 0) x (0, 0, -1) in component "DXF Export"
  line L0 (-17.35, 5.2) -> (-17.35, 9.2)
  line L1 (-17.35, 9.2) -> (-12.85, 9.2)
  line L2 (-12.85, 9.2) -> (-12.85, 5.2)
  line L3 (-12.85, 5.2) -> (-17.35, 5.2)
  line L4 (-0.8, 25.4) -> (-21.2, 25.4)
  line L5 (-21.2, 25.4) -> (-21.2, 29.4)
  line L6 (-21.2, 29.4) -> (-25.7, 29.4)
  line L7 (-25.7, 29.4) -> (-25.7, 25.4)
  line L8 (-25.7, 25.4) -> (-30.2, 25.4)
  line L9 (-30.2, 25.4) -> (-30.2, 20.9)
  line L10 (-30.2, 13.5) -> (-29.3, 13.5)
  line L11 (-29.3, 13.5) -> (-29.3, 14.2)
  line L12 (-29.3, 14.2) -> (-28.1, 14.2)
  line L13 (-28.1, 14.2) -> (-28.1, 11.2)
  line L14 (-28.1, 11.2) -> (-29.3, 11.2)
  line L15 (-29.3, 11.2) -> (-29.3, 11.9)
  line L16 (-29.3, 11.9) -> (-30.2, 11.9)
  line L17 (-30.2, 11.9) -> (-30.2, 9)
  line L18 (-30.2, 9) -> (-34.2, 9)
  line L19 (-34.2, 9) -> (-34.2, 4.5)
  line L20 (-34.2, 4.5) -> (-30.2, 4.5)
  line L21 (-30.2, 4.5) -> (-30.2, 0)
  line L22 (-30.2, 0) -> (-25.7, 0)
  line L23 (-25.7, 0) -> (-25.7, -4)
  line L24 (-25.7, -4) -> (-21.2, -4)
  line L25 (-21.2, -4) -> (-21.2, 0)
  line L26 (-21.2, 0) -> (-0.8, 0)
  line L27 (-0.8, 0) -> (-0.8, 0.9)
  line L28 (-0.8, 0.9) -> (-1.5, 0.9)
  line L29 (-1.5, 0.9) -> (-1.5, 2.1)
  line L30 (-1.5, 2.1) -> (1.5, 2.1)
  line L31 (1.5, 2.1) -> (1.5, 0.9)
  line L32 (1.5, 0.9) -> (0.8, 0.9)
  line L33 (0.8, 0.9) -> (0.8, 0)
  line L34 (0.8, 0) -> (21.2, 0)
  line L35 (21.2, 0) -> (21.2, -4)
  line L36 (21.2, -4) -> (25.7, -4)
  line L37 (25.7, -4) -> (25.7, 0)
  line L38 (25.7, 0) -> (30.2, 0)
  line L39 (30.2, 0) -> (30.2, 4.5)
  line L40 (30.2, 4.5) -> (34.2, 4.5)
  line L41 (34.2, 4.5) -> (34.2, 9)
  line L42 (34.2, 9) -> (30.2, 9)
  line L43 (30.2, 9) -> (30.2, 11.9)
  line L44 (30.2, 11.9) -> (29.3, 11.9)
  line L45 (29.3, 11.9) -> (29.3, 11.2)
  line L46 (29.3, 11.2) -> (28.1, 11.2)
  line L47 (28.1, 11.2) -> (28.1, 14.2)
  line L48 (28.1, 14.2) -> (29.3, 14.2)
  line L49 (29.3, 14.2) -> (29.3, 13.5)
  line L50 (29.3, 13.5) -> (30.2, 13.5)
  line L51 (30.2, 13.5) -> (30.2, 16.4)
  line L52 (30.2, 25.4) -> (25.7, 25.4)
  line L53 (25.7, 25.4) -> (25.7, 29.4)
  line L54 (25.7, 29.4) -> (21.2, 29.4)
  line L55 (21.2, 29.4) -> (21.2, 25.4)
  line L56 (21.2, 25.4) -> (0.8, 25.4)
  line L57 (0.8, 25.4) -> (0.8, 24.5)
  line L58 (0.8, 24.5) -> (1.5, 24.5)
  line L59 (1.5, 24.5) -> (1.5, 23.3)
  line L60 (1.5, 23.3) -> (-1.5, 23.3)
  line L61 (-1.5, 23.3) -> (-1.5, 24.5)
  line L62 (-1.5, 24.5) -> (-0.8, 24.5)
  line L63 (-0.8, 24.5) -> (-0.8, 25.4)
  line L64 (-30.2, 20.9) -> (-34.2, 20.9)
  line L65 (-34.2, 20.9) -> (-34.2, 16.4)
  line L66 (-34.2, 16.4) -> (-30.2, 16.4)
  line L67 (-30.2, 16.4) -> (-30.2, 13.5)
  line L68 (30.2, 16.4) -> (34.2, 16.4)
  line L69 (34.2, 16.4) -> (34.2, 20.9)
  line L70 (34.2, 20.9) -> (30.2, 20.9)
  line L71 (30.2, 20.9) -> (30.2, 25.4)
sketch "Left" plane through (-24.2, 0, 0) normal (-1, 0, 0) x (0, 0, 1) in component "DXF Export"
  line L0 (-12.85, 9.2) -> (-12.85, 5.2)
  line L1 (-12.85, 5.2) -> (-17.35, 5.2)
  line L2 (-17.35, 5.2) -> (-17.35, 9.2)
  line L3 (-17.35, 9.2) -> (-12.85, 9.2)
  line L4 (25.7, -4) -> (25.7, 0)
  line L5 (25.7, 0) -> (30.2, 0)
  line L6 (30.2, 0) -> (30.2, 4.5)
  line L7 (30.2, 4.5) -> (34.2, 4.5)
  line L8 (34.2, 4.5) -> (34.2, 9)
  line L9 (34.2, 9) -> (30.2, 9)
  line L10 (30.2, 9) -> (30.2, 11.9)
  line L11 (30.2, 11.9) -> (29.3, 11.9)
  line L12 (29.3, 11.9) -> (29.3, 11.2)
  line L13 (29.3, 11.2) -> (28.1, 11.2)
  line L14 (28.1, 11.2) -> (28.1, 14.2)
  line L15 (28.1, 14.2) -> (29.3, 14.2)
  line L16 (29.3, 14.2) -> (29.3, 13.5)
  line L17 (29.3, 13.5) -> (30.2, 13.5)
  line L18 (30.2, 13.5) -> (30.2, 16.4)
  line L19 (30.2, 25.4) -> (25.7, 25.4)
  line L20 (25.7, 25.4) -> (25.7, 29.4)
  line L21 (25.7, 29.4) -> (21.2, 29.4)
  line L22 (21.2, 29.4) -> (21.2, 25.4)
  line L23 (21.2, 25.4) -> (0.8, 25.4)
  line L24 (0.8, 25.4) -> (0.8, 24.5)
  line L25 (0.8, 24.5) -> (1.5, 24.5)
  line L26 (1.5, 24.5) -> (1.5, 23.3)
  line L27 (1.5, 23.3) -> (-1.5, 23.3)
  line L28 (-1.5, 23.3) -> (-1.5, 24.5)
  line L29 (-1.5, 24.5) -> (-0.8, 24.5)
  line L30 (-0.8, 24.5) -> (-0.8, 25.4)
  line L31 (-0.8, 25.4) -> (-21.2, 25.4)
  line L32 (-21.2, 25.4) -> (-21.2, 29.4)
  line L33 (-21.2, 29.4) -> (-25.7, 29.4)
  line L34 (-25.7, 29.4) -> (-25.7, 25.4)
  line L35 (-25.7, 25.4) -> (-30.2, 25.4)
  line L36 (-30.2, 25.4) -> (-30.2, 20.9)
  line L37 (-30.2, 13.5) -> (-29.3, 13.5)
  line L38 (-29.3, 13.5) -> (-29.3, 14.2)
  line L39 (-29.3, 14.2) -> (-28.1, 14.2)
  line L40 (-28.1, 14.2) -> (-28.1, 11.2)
  line L41 (-28.1, 11.2) -> (-29.3, 11.2)
  line L42 (-29.3, 11.2) -> (-29.3, 11.9)
  line L43 (-29.3, 11.9) -> (-30.2, 11.9)
  line L44 (-30.2, 11.9) -> (-30.2, 9)
  line L45 (-30.2, 9) -> (-34.2, 9)
  line L46 (-34.2, 9) -> (-34.2, 4.5)
  line L47 (-34.2, 4.5) -> (-30.2, 4.5)
  line L48 (-30.2, 4.5) -> (-30.2, 0)
  line L49 (-30.2, 0) -> (-25.7, 0)
  line L50 (-25.7, 0) -> (-25.7, -4)
  line L51 (-25.7, -4) -> (-21.2, -4)
  line L52 (-21.2, -4) -> (-21.2, 0)
  line L53 (-21.2, 0) -> (-0.8, 0)
  line L54 (-0.8, 0) -> (-0.8, 0.9)
  line L55 (-0.8, 0.9) -> (-1.5, 0.9)
  line L56 (-1.5, 0.9) -> (-1.5, 2.1)
  line L57 (-1.5, 2.1) -> (1.5, 2.1)
  line L58 (1.5, 2.1) -> (1.5, 0.9)
  line L59 (1.5, 0.9) -> (0.8, 0.9)
  line L60 (0.8, 0.9) -> (0.8, 0)
  line L61 (0.8, 0) -> (21.2, 0)
  line L62 (21.2, 0) -> (21.2, -4)
  line L63 (21.2, -4) -> (25.7, -4)
  line L64 (30.2, 16.4) -> (34.2, 16.4)
  line L65 (34.2, 16.4) -> (34.2, 20.9)
  line L66 (34.2, 20.9) -> (30.2, 20.9)
  line L67 (30.2, 20.9) -> (30.2, 25.4)
  line L68 (-30.2, 20.9) -> (-34.2, 20.9)
  line L69 (-34.2, 20.9) -> (-34.2, 16.4)
  line L70 (-34.2, 16.4) -> (-30.2, 16.4)
  line L71 (-30.2, 16.4) -> (-30.2, 13.5)
sketch "Mid Plane" plane through (0, 9.2, 0) normal (0, 1, 0) x (-1, 0, 0) in component "DXF Export"
  line L0 (20.2, 30.2) -> (12.35, 30.2)
  line L1 (12.35, 30.2) -> (12.35, 34.2)
  line L2 (12.35, 34.2) -> (7.85, 34.2)
  line L3 (7.85, 34.2) -> (7.85, 30.2)
  line L4 (7.85, 30.2) -> (-20.2, 30.2)
  line L5 (-20.2, 30.2) -> (-20.2, 17.35)
  line L6 (-20.2, 17.35) -> (-24.2, 17.35)
  line L7 (-24.2, 17.35) -> (-24.2, 12.85)
  line L8 (-24.2, 12.85) -> (-20.2, 12.85)
  line L9 (-20.2, 12.85) -> (-20.2, -30.2)
  line L10 (-20.2, -30.2) -> (-12.35, -30.2)
  line L11 (-12.35, -30.2) -> (-12.35, -34.2)
  line L12 (-12.35, -34.2) -> (-7.85, -34.2)
  line L13 (-7.85, -34.2) -> (-7.85, -30.2)
  line L14 (-7.85, -30.2) -> (20.2, -30.2)
  line L15 (20.2, -30.2) -> (20.2, -17.35)
  line L16 (20.2, -17.35) -> (24.2, -17.35)
  line L17 (24.2, -17.35) -> (24.2, -12.85)
  line L18 (24.2, -12.85) -> (20.2, -12.85)
  line L19 (20.2, -12.85) -> (20.2, 30.2)
equation "d1 = object_length"
equation "d2 = object_width"
equation "d3 = tolerance_to_object"
equation "d4 = material_thickness + tolerance_to_object"
equation "d19 = object_height + tolerance_to_object * 2"
equation "d161 = 68.40 mm / 6"
equation "d199 = 4 mm"
equation "d210 = d199"
equation "d232 = d199"
equation "object_height = 20 mm"
equation "object_width = 25.57 mm"
equation "object_length = 52 mm"
equation "tolerance_to_object = 0.5 mm"
equation "pin_thickness = 4.5 mm"